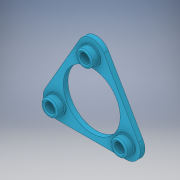
# Autodesk Inventor part: Bottom
Saved by Autodesk Inventor 2019.1 (Build 231200000, 200)
## iProperties
Created: 2019-01-01
Part Number: Bottom
Material: Generisch
Document SubType Name: Modeling
Designer: JochenAlt
Density: 1 g/cm^3
Appearance: Vorgabe
Author: JochenAlt
Autodesk Inventor part; units mm, degrees
ref_plane "YZ Plane" through (0, 0, 0) normal (1, 0, 0) x (0, 1, 0)
ref_plane "XZ Plane" through (0, 0, 0) normal (0, 1, 0) x (-1, 0, 0)
ref_plane "XY Plane" through (0, 0, 0) normal (0, 0, 1) x (1, 0, 0)
sketch "Skizze1" plane through (0, 0, 0) normal (0, 0, 1) x (1, 0, 0)
  circle A0 centre (0, 0) radius 17.15 construction
  line L0 (0, 31.15) -> (0, -25.2) construction
  circle A1 centre (0, 17.15) radius 2.1
  circle A2 centre (14.8523, -8.575) radius 2.1
  circle A3 centre (-14.8523, -8.575) radius 2.1
  line L1 (0, 17.15) -> (14.8523, -8.575) construction
  line L2 (-14.8523, -8.575) -> (14.8523, -8.575) construction
  line L3 (-14.8523, -8.575) -> (0, 17.15) construction
  line L4 (5.1529, 20.125) -> (20.0052, -5.6)
  line L5 (14.8523, -14.525) -> (-14.8523, -14.525)
  line L6 (-20.0052, -5.6) -> (-5.1529, 20.125)
  arc A4 (-20.0052, -5.6) -> (-14.8523, -14.525) centre (-14.8523, -8.575) ccw
  arc A5 (14.8523, -14.525) -> (20.0052, -5.6) centre (14.8523, -8.575) ccw
  arc A6 (5.1529, 20.125) -> (-5.1529, 20.125) centre (0, 17.15) ccw
  circle A7 centre (0, 17.15) radius 3.45
  circle A8 centre (-14.8523, -8.575) radius 3.45
  circle A9 centre (14.8523, -8.575) radius 3.45
  circle A10 centre (0, 17.15) radius 3.95
  circle A11 centre (14.8523, -8.575) radius 3.95
  circle A12 centre (-14.8523, -8.575) radius 3.95
  circle A13 centre (0, 0) radius 12.2
  point P0 (0, 13.2)
  point P1 (0, 12.2)
  dimension "d1" = 4.2
  dimension "d2" = 17.15
  dimension "d3" = 0.5
  dimension "d4" = 6.9
  dimension "d5" = 2
  dimension "d12" = 1
  constraints: 12 centre point, 12 end point, 11 coincident, 9 point on circle, 7 equal radius, 6 tangent, 3 point on line, 2 equal length, 2 vertical alignment, 5 other
  measures "d1" diameter of A1
  measures "d2" radius of A0
  measures "d4" diameter of A7
  measures "d12" distance of point (0, 12.2) point (0, 13.2)
extrude "Extrusion1" add sketch "Skizze1" along normal blind 2 contours L4 A5 L5 A4 L6 A6 | A7 | A8 | A9 | A10 | A11 | A12
extrude "Extrusion2" add sketch "Skizze1" along normal blind 0.5 from surface at 2 contours A7 | A8 | A9 | A10 | A11 | A12
extrude "Extrusion3" add sketch "Skizze1" along normal blind 3 from surface at 2.5 contours A7 | A8 | A9
chamfer "Fase1" distance 0.5 angle 45 6 edges at (-3.45, 17.15, 5.5) (-18.3023, -8.575, 5.5) (11.4023, -8.575, 5.5) (-2.1, 17.15, 5.5) (-16.9523, -8.575, 5.5) (12.7523, -8.575, 5.5)
